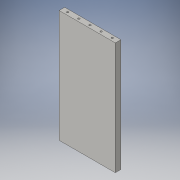
# Autodesk Inventor part: bottom
Saved by Autodesk Inventor 2016 (Build 200138000, 138)
## iProperties
Created: 2015-09-30
Part Number: bottom
Material: Generic
Document SubType Name: Modeling
Designer: Jesse Stevenson
Density: 1 g/cm^3
Appearance: Default
Author: Jesse Stevenson
Autodesk Inventor part; units mm, degrees
ref_plane "YZ Plane" through (0, 0, 0) normal (1, 0, 0) x (0, 1, 0)
ref_plane "XZ Plane" through (0, 0, 0) normal (0, 1, 0) x (-1, 0, 0)
ref_plane "XY Plane" through (0, 0, 0) normal (0, 0, 1) x (1, 0, 0)
sketch "Sketch1" plane through (0, 0, 0) normal (0, 0, 1) x (1, 0, 0)
  line L0 (0, 0) -> (63.9572, 0)
  line L1 (63.9572, 0) -> (63.9572, 128.0414)
  line L2 (63.9572, 128.0414) -> (0, 128.0414)
  line L3 (0, 128.0414) -> (0, 0)
  dimension "d0" = 63.9572
  dimension "d1" = 128.0414
  constraints: 8 end point, 2 parallel, 1 horizontal, 1 perpendicular
  measures "d0" distance of L2.end L1.end
  measures "d1" distance of L1.end L0.end
extrude "Extrusion1" add sketch "Sketch1" along normal blind 6.35
sketch "Sketch2" plane through (0, 128.0414, 0) normal (0, 1, 0) x (1, 0, 0)
  line L0 (63.9572, 0) -> (0, 0) construction
  line L1 (0, 0) -> (0, -6.35) construction
  line L2 (63.9572, -6.35) -> (0, -6.35) construction
  line L3 (63.9572, 0) -> (63.9572, -6.35) construction
  line L4 (0, -6.35) -> (63.9572, -6.35) construction
  line L5 (31.9786, -6.35) -> (31.9786, 0) construction
  circle A0 centre (31.9786, -3.175) radius 1.0541
  dimension "d4" = 2.1082
  constraints: 3 midpoint, 2 end point, 1 centre point
  measures "d4" diameter of A0
extrude "Extrusion2" cut sketch "Sketch2" against normal blind 6.35
pattern_linear "Rectangular Pattern1" count 3 spacing 12.7 along (-1, 0, 0) count 3 spacing 12.7 along (1, 0, 0) of "Extrusion2"
body "Solid1"
